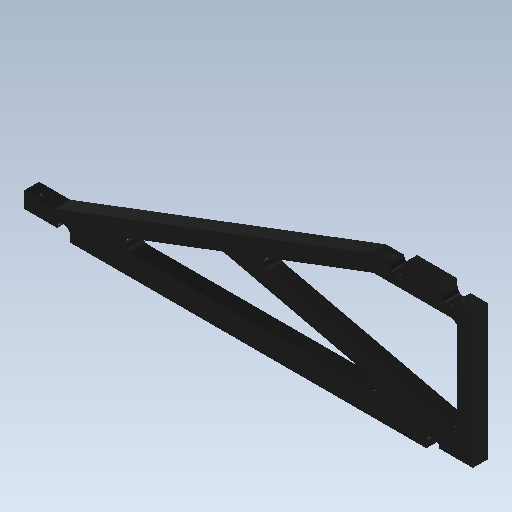
# Autodesk Inventor part: ForeArm_diagonal
Saved by Autodesk Inventor 2020 (Build 240168000, 168)
## iProperties
Created: 2016-05-04
Part Number: ForeArm_diagonal
Material: アセタール樹脂、黒
Document SubType Name: Modeling
Designer: hiroaki
Density: 1.425 g/cm^3
Appearance: 滑らか - 黒
Mass: 16.6114 g
Surface Area: 81.8888 cm^2
Volume: 11.6571 cm^3
Description: POM T5
Author: hiroaki
Autodesk Inventor part; units mm, degrees
ref_plane "YZ Plane" through (0, 0, 0) normal (1, 0, 0) x (0, 1, 0)
ref_plane "XZ Plane" through (0, 0, 0) normal (0, 1, 0) x (-1, 0, 0)
ref_plane "XY Plane" through (0, 0, 0) normal (0, 0, 1) x (1, 0, 0)
sketch "スケッチ1" plane through (0, 0, 0) normal (0, 0, 1) x (1, 0, 0)
  line L0 (-72.5, -21.75) -> (72.5, -21.75) construction
  line L1 (72.5, -21.75) -> (72.5, 21.75) construction
  line L2 (72.5, 21.75) -> (-72.5, 21.75) construction
  line L3 (-72.5, 21.75) -> (-72.5, -21.75) construction
  line L4 (-72.5, -21.75) -> (72.5, 21.75) construction
  line L5 (72.5, -21.75) -> (-72.5, 21.75) construction
  line L6 (-67.5, 21.75) -> (-67.5, -21.75) construction
  line L7 (0, 0) -> (0, 21.75) construction
  line L8 (0, 0) -> (-72.5, 0) construction
  line L9 (67.5, 21.75) -> (67.5, -11.6593) construction
  line L10 (-72.5, -21.75) -> (-61.7, -21.75)
  line L11 (49.5, 21.75) -> (49.5, 23.75)
  line L12 (49.5, 23.75) -> (62.5, 23.75)
  line L13 (62.5, 23.75) -> (62.5, 21.75)
  line L14 (66.7, 21.75) -> (72.5, 21.75)
  line L15 (72.5, 21.75) -> (72.5, -21.75)
  line L16 (72.5, -21.75) -> (61.7, -21.75)
  line L17 (-57.5, -21.75) -> (-57.5, -23.75)
  line L18 (-57.5, -23.75) -> (57.5, -23.75)
  line L19 (57.5, -23.75) -> (57.5, -21.75)
  arc A0 (45.3, 21.75) -> (49.5, 21.75) centre (47.4, 21.75) ccw
  arc A1 (62.5, 21.75) -> (66.7, 21.75) centre (64.6, 21.75) ccw
  arc A2 (-57.5, -21.75) -> (-61.7, -21.75) centre (-59.6, -21.75) ccw
  arc A3 (61.7, -21.75) -> (57.5, -21.75) centre (59.6, -21.75) ccw
  line L20 (-72.5, -21.75) -> (-72.5, -16.75)
  line L21 (45.3, 21.75) -> (39.5, 21.75)
  line L22 (66.95, 24.476) -> (70.05, 24.476) construction
  line L23 (70.05, 24.476) -> (70.05, 13.3235) construction
  line L24 (70.05, 13.3235) -> (66.95, 13.3235) construction
  line L25 (66.95, 13.3235) -> (66.95, 24.476) construction
  line L26 (68.5, 24.476) -> (68.5, 13.3235) construction
  line L27 (41.95, 24.476) -> (45.05, 24.476) construction
  line L28 (45.05, 24.476) -> (45.05, 13.9945) construction
  line L29 (45.05, 13.9945) -> (41.95, 13.9945) construction
  line L30 (41.95, 13.9945) -> (41.95, 24.476) construction
  line L31 (43.5, 24.476) -> (43.5, 13.9945) construction
  line L32 (-72.5, -16.75) -> (-62.8649, -16.75)
  line L33 (-62.1586, -16.6211) -> (39.5, 21.75)
  line L34 (40.0708, 16.6211) -> (6.3776, 3.9036) construction
  line L35 (-48.341, -16.75) -> (67.5, -16.75) construction
  line L36 (67.5, -16.75) -> (67.5, 14.75) construction
  line L37 (65.5, 16.75) -> (40.7771, 16.75)
  line L38 (67.5, -16.75) -> (-3.9644, 0) construction
  line L39 (-8.731, -1.7991) -> (-38.085, -12.8789)
  line L40 (-7.5683, -1.7231) -> (39.7036, -12.8028)
  line L41 (39.2472, -16.75) -> (-37.3787, -16.75)
  line L42 (6.6274, 0.0852) -> (65.0436, -13.6065)
  line L43 (67.5, -14.1822) -> (67.5, 16.75)
  arc A4 (65.0436, -13.6065) -> (67.5, -11.6593) centre (65.5, -11.6593) ccw
  arc A5 (6.3776, 3.9036) -> (6.6274, 0.0852) centre (7.0838, 2.0324) ccw
  line L44 (40.0708, 16.6211) -> (6.3776, 3.9036)
  arc A6 (40.7771, 16.75) -> (40.0708, 16.6211) centre (40.7771, 14.75) ccw
  arc A7 (67.5, 14.75) -> (65.5, 16.75) centre (65.5, 14.75) ccw
  arc A8 (-38.085, -12.8789) -> (-37.3787, -16.75) centre (-37.3787, -14.75) ccw
  arc A9 (-7.5683, -1.7231) -> (-8.731, -1.7991) centre (-8.0247, -3.6703) ccw
  arc A10 (39.2472, -16.75) -> (39.7036, -12.8028) centre (39.2472, -14.75) ccw
  arc A11 (-62.8649, -16.75) -> (-62.1586, -16.6211) centre (-62.8649, -14.75) ccw
  point P0 (67.5, -21.75)
  point P1 (-62.5, -16.75)
  point P2 (40.4122, 16.75)
  point P3 (-8.1612, -1.5841)
  point P4 (56.5446, -16.75)
  point P5 (67.5, -11.6593)
  dimension "d16" = 5
  dimension "d20" = 43.5
  dimension "d40" = 135
  dimension "d41" = 10
  dimension "d42" = 2.1
  dimension "d43" = 2
  dimension "d44" = 5
  dimension "d45" = 10
  dimension "d46" = 10
  dimension "d48" = 3.1
  dimension "d50" = 4
  dimension "d51" = 25
  dimension "d52" = 3.1
  dimension "d62" = 6
  dimension "d63" = 6
  dimension "d88" = 10
  dimension "d90" = 5
  dimension "d91" = 5
  dimension "d93" = 5
  dimension "d94" = 94.8651
  dimension "d96" = 47.4325
  dimension "d97" = 2.5
  dimension "d98" = 5
  dimension "d99" = 2
  dimension "d100" = 2
  dimension "d101" = 5
  dimension "d102" = 2
  dimension "d103" = 2
  dimension "d104" = 2
  dimension "d105" = 2
  constraints: 90 end point, 27 point on line, 24 point on circle, 19 tangent, 14 perpendicular, 12 centre point, 10 parallel, 8 collinear, 8 midpoint, 5 equal radius, 5 horizontal, 4 horizontal alignment, 2 symmetric about line, 2 vertical, 3 other
  measures "d16" distance between parallel lines of L3 L6
  measures "d20" distance of L2.end L0.start
  measures "d40" distance between parallel lines of L9 L6
  measures "d41" distance between parallel lines of L6 L17
  measures "d42" radius of A2
  measures "d43" distance between parallel lines of L0 L18
  measures "d44" distance from line of L10 L20.end
  measures "d45" distance between parallel lines of L1 L13
  measures "d46" distance from line of L21.end L11
  measures "d48" distance of L22.start L22.end
  measures "d50" distance between parallel lines of L1 L26
  measures "d51" distance between parallel lines of L26 L31
  measures "d52" distance of L27.start L27.end
  measures "d62" distance between parallel lines of L13 L26
  measures "d63" distance between parallel lines of L31 L11
  measures "d88" distance of L20.end point (-62.5, -16.75)
  measures "d90" distance between parallel lines of L33 L34
  measures "d91" distance between parallel lines of L1 L36
  measures "d93" distance between parallel lines of L16 L35
  measures "d94" distance of point (40.412, 16.75) L35.start
  measures "d96" distance of L38.end point (40.412, 16.75)
  measures "d97" distance between parallel lines of L40 L38
  measures "d98" distance between parallel lines of L40 L42
  measures "d99" radius of A4
  measures "d100" radius of A5
  measures "d101" distance between parallel lines of L37 L2
  measures "d102" radius of A6
  measures "d103" radius of A7
  measures "d104" radius of A8
  measures "d105" radius of A11
extrude "押し出し1" add sketch "スケッチ1" along normal blind 2.5
mirror "ミラー1" about plane through (0, 0, 0) normal (0, 0, -1) of "押し出し1"
sketch "スケッチ2" plane through (-72.5, -21.75, 2.5) normal (0, -1, 0) x (1, 0, 0)
  line L0 (0, -5) -> (0, 0)
  line L1 (15, -5) -> (130, -5) construction
  line L2 (72.5, -5) -> (72.5, 0) construction
  line L3 (15, 0) -> (130, 0) construction
  point P0 (72.5, -2.5)
  point P1 (140, -2.5)
  point P2 (0, -2.5)
  constraints: 4 end point, 3 midpoint
hole "穴1" at (67.5, -21.75, 0) direction (0, 1, 0) diameter 2.459 depth 2 thread size "M3x0.5" class "6H" standard "ISO Metric profile"
sketch "スケッチ4" plane through (66.7, 21.75, 2.5) normal (0, 1, 0) x (1, 0, 0)
  line L0 (5.8, 5) -> (5.8, 0) projected
  point P0 (-66.7, 2.5)
  point P1 (1.8, 2.5)
  point P2 (-23.2, 2.5)
  point P3 (5.8, 2.5)
  dimension "d53" = 4
  dimension "d54" = 25
  constraints: 2 horizontal alignment, 1 midpoint
  measures "d53" distance from line of point (1.8, 2.5) L0
  measures "d54" distance of point (-23.2, 2.5) point (1.8, 2.5)
hole "穴2" at (68.5, 21.75, 0) at (43.5, 21.75, 0) direction (0, -1, 0) diameter 2.459 depth 2.5 thread size "M3x0.5" class "6H" standard "ISO Metric profile"
sketch "スケッチ7" plane through (-72.5, -21.75, 2.5) normal (0, -1, 0) x (1, 0, 0)
  line L0 (0, -5) -> (0, 0) projected
  line L1 (15, 0) -> (130, 0) projected
  line L2 (15, -5) -> (130, -5) projected
  line L3 (0, -2.5) -> (5, -2.5)
  point P0 (72.5, -2.5)
  dimension "d80" = 5
  constraints: 2 end point, 1 horizontal, 1 midpoint
  measures "d80" distance from line of L3.end L0
hole "穴3" at (-67.5, -21.75, 0) direction (0, 1, 0) diameter 3 end through all
equation "\"d16\" = d4"
equation "\"d40\" = d6"
equation "\"d41\" = d3"
equation "\"d46\" = d45"
equation "\"d63\" = d62"
equation "\"d53\" = d50"
equation "\"d54\" = d51"
equation "\"d4\" = 5"
equation "\"d6\" = 135"
equation "\"d3\" = 10"
